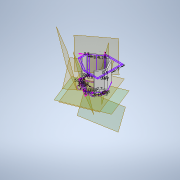
# Autodesk Inventor part: mouse_cam_base_final_withgyro_wall
Saved by Autodesk Inventor 2022 (Build 260153000, 153)
## iProperties
Created: 2022-03-01
Part Number: mouse_cam_base_final_withgyro_wall
Material: Generic
Document SubType Name: Modeling
Designer: Cornell
Density: 1 g/cm^3
Appearance: Default
Author: Cornell
Autodesk Inventor part; units mm, degrees
sketch "Sketch1" plane through (0, 0, 0) normal (0, 1, 0) x (-1, 0, 0)
  line L0 (0, 0) -> (0, 6.2) construction
  line L1 (0, 6.2) -> (10.144349, 0.343157) construction
  line L2 (0, 0) -> (-2.7, 0) construction
  line L3 (-2.7, 0) -> (-2.7, 5.13) construction
  line L4 (-2.7, 5.13) -> (0, 6.2) construction
  line L5 (-2.7, 0) -> (-5.7, 0) construction
  line L6 (-5.7, 0) -> (-2.7, 5.13) construction
  line L7 (-5.7, 0) -> (-6.5, 0)
  line L8 (-6.423049, 0.342344) -> (-3.493848, 5.594239)
  line L9 (0.128209, 7.130954) -> (-3.493848, 5.594239) construction
  line L10 (0.128209, 7.130954) -> (10.551194, 1.035641) construction
  line L11 (10.144349, 0.343157) -> (0, 6.2) construction
  line L12 (-5.7, 0) -> (-2.7, 5.13) construction
  line L13 (0, 6.2) -> (10.144349, 0.343157) construction
  line L14 (10.551194, 1.035641) -> (10.144349, 0.343157) construction
  line L15 (0, 6.2) -> (0.438353, 6.949583)
  line L16 (0.438353, 6.949583) -> (3.02804, 5.435146) construction
  line L17 (3.02804, 5.435146) -> (2.602221, 4.697607) construction
  line L18 (0, 6.2) -> (-0.381289, 6.498511) construction
  line L19 (-0.381289, 6.498511) -> (0.106711, 7.121833) construction
  line L20 (-5.7, 0) -> (-2.7, -5.13) construction
  line L21 (-6.423049, -0.342344) -> (-3.493848, -5.594239)
  line L22 (-6.423049, 0.342344) -> (-6.423049, -0.342344)
  line L23 (-5.559009, 0.241095) -> (-5.559009, -0.241095)
  line L24 (-5.559009, 0) -> (4.440991, 0) construction
  line L25 (-5.559009, 0) -> (5.440991, 0) construction
  line L26 (5.440991, 0) -> (6.440991, 0) construction
  line L27 (5.440991, 0) -> (6.240991, 0)
  line L28 (10.144349, 0.343157) -> (10.144349, -0.005356)
  line L29 (10.144349, -0.005356) -> (10.144349, -0.347701)
  line L30 (10.144349, -0.347701) -> (5.339701, -3.117122) construction
  line L31 (10.551194, 1.035641) -> (10.551194, -1.035641) construction
  line L32 (10.551194, -1.035641) -> (6.240991, -3.556227) construction
  line L33 (5.440991, 0) -> (7.810991, 0) construction
  line L34 (7.810991, 0) -> (7.810991, 1.690322)
  line L35 (7.810991, 0) -> (7.810991, -1.692659)
  line L36 (7.810991, 0) -> (8.610991, 0) construction
  line L37 (8.610991, 0) -> (8.610991, 1.228442)
  line L38 (8.610991, 0) -> (8.610991, -1.231535)
  line L39 (8.610991, -1.231535) -> (8.610991, -2.170262)
  line L40 (7.810991, -1.692659) -> (7.810991, -2.638099)
  line L41 (0, -6.2) -> (0, -4.7)
  line L42 (6.240991, -3.556227) -> (2.598076, -5.686587) construction
  line L43 (-2.951462, -4.7) -> (-5.559009, -0.241095)
  line L44 (-3.493848, -5.594239) -> (-2.951462, -4.7)
  line L45 (-5.559009, 0.241095) -> (-2.951462, 4.7)
  line L46 (10.551194, 1.035641) -> (2.755992, 5.594239) construction
  line L47 (2.602221, 4.697607) -> (10.144349, 0.343157) construction
  line L48 (-5.559009, -0.241095) -> (-5.559009, 0.241095)
  line L49 (-2.951462, 4.7) -> (-3.493848, 5.594239)
  line L50 (-6.423049, -0.342344) -> (-5.559009, -0.241095)
  line L51 (-6.423049, 0.342344) -> (-5.559009, 0.241095)
  line L52 (7.810991, -1.692659) -> (8.610991, -1.231535)
  line L53 (7.810991, 1.690322) -> (8.610991, 1.228442)
  line L54 (8.610991, 1.228442) -> (8.610991, 2.170262)
  line L55 (7.810991, 1.690322) -> (7.810991, 2.638099)
  line L56 (7.810991, 2.638099) -> (8.610991, 2.170262)
  line L57 (2.593853, -4.401195) -> (-2.951462, -4.7)
  line L58 (-3.493848, -5.594239) -> (2.69542, -5.260734)
  line L59 (2.593853, -4.401195) -> (8.610991, -1.231535)
  line L60 (2.69542, -5.260734) -> (8.610991, -2.170262)
  line L61 (2.593853, -4.401195) -> (2.69542, -5.260734)
  line L62 (2.593853, 4.401195) -> (-2.951462, 4.7)
  line L63 (-3.493848, 5.594239) -> (2.69542, 5.260734)
  line L64 (2.593853, 4.401195) -> (2.69542, 5.260734)
  line L65 (-2.951462, 4.7) -> (2.593853, 4.401195)
  line L66 (2.644637, 4.830965) -> (2.69542, 5.260734)
  line L67 (-3.493848, 5.594239) -> (-2.951462, 4.7)
  point P0 (2.602221, 4.697607)
  point P1 (-5.29708, 0.688993)
  dimension "d0" = 6.2
  dimension "d1" = 60
  dimension "d2" = 2.7
  dimension "d3" = 5.13
  dimension "d4" = 3
  dimension "d7" = 0.8
  dimension "d8" = 0.8
  dimension "d20" = 3
  dimension "d33" = 10
  dimension "d36" = 0.8
  dimension "d73" = 2.37
  dimension "d74" = 0.8
  constraints: 136 end point, 28 point on line, 14 collinear, 7 perpendicular, 7 symmetric about line, 4 parallel, 4 vertical, 3 horizontal, 2 midpoint
  measures "d0" distance of L0.start L0.end
  measures "d1" angle of L0 L1
  measures "d2" distance of L0.start L2.end
  measures "d3" distance of L2.end L3.end
  measures "d4" distance of L2.end L5.end
  measures "d7" distance of L5.end L7.end
  measures "d8" distance of L5.end L8.start
  measures "d20" distance of L15.end L16.end
  measures "d33" distance of L24.start L24.end
  measures "d36" distance of L25.end L27.end
  measures "d73" distance of L25.end L33.end
  measures "d74" distance of L33.end L36.end
ref_plane "Work Plane1" through (2.7, 0, 5.13) normal (0, 1, 0) x (-0.9296593, 0, 0.3684205)
ref_plane "Work Plane2" through (2.7, 3, 5.13) normal (0, 1, 0) x (-0.9296593, 0, 0.3684205)
sketch "Sketch2" plane through (2.7, 3, 5.13) normal (0, 1, 0) x (-0.9296593, 0, 0.3684205)
  line L0 (-5.025918, -0.734007) -> (-6.376038, -1.814103)
  line L1 (-5.876282, -2.438798) -> (-1.068891, 1.407115)
  line L2 (3.395875, 2.207115) -> (-1.349515, 2.207115)
  line L3 (-1.349515, 2.207115) -> (-5.025918, -0.734007)
  line L4 (0.620083, -5.763887) -> (-1.890319, -4.77089) construction
  line L5 (-6.938992, -5.570456) -> (-7.184919, -3.859038)
  line L6 (-6.393053, -3.745249) -> (-5.517376, -9.839118)
  line L7 (-5.517376, -9.839118) -> (-2.260723, -12.893351)
  line L8 (-2.260723, -12.893351) -> (-2.807982, -13.476881)
  line L9 (-2.807982, -13.476881) -> (-6.269327, -10.230679)
  line L10 (-6.269327, -10.230679) -> (-6.938992, -5.570456)
  line L11 (-5.876282, -2.438798) -> (-6.393053, -3.745249)
  line L12 (-7.184919, -3.859038) -> (-6.376038, -1.814103)
  line L13 (-2.260723, -12.893351) -> (-1.956037, -13.211044)
  line L14 (-2.807982, -13.476881) -> (-2.146425, -14.097318)
  line L15 (6.305657, -10.853277) -> (-1.956037, -13.211044)
  line L16 (6.901194, -11.51526) -> (-2.146425, -14.097318)
  line L17 (-1.349515, 2.207115) -> (-2.349515, 1.407115)
  line L18 (-5.646461, -8.940808) -> (-6.438327, -9.054598)
  line L19 (6.901194, -11.51526) -> (7.800754, -11.250894)
  line L20 (6.667165, -11.582048) -> (8.800527, -6.188688)
  line L21 (7.800754, -11.250894) -> (9.479308, -7.007336)
  line L22 (6.305657, -10.853277) -> (8.171706, -10.31309)
  line L23 (9.451627, -6.973952) -> (9.479308, -7.007336)
  line L24 (9.479308, -7.007336) -> (9.191715, -7.734401)
  line L25 (9.191715, -7.734401) -> (9.479308, -7.007336)
  line L26 (9.479308, -7.007336) -> (8.800527, -6.188688)
  line L27 (-1.068891, 1.407115) -> (-1.349515, 2.207115)
  line L28 (4.0365, -0.443004) -> (3.982037, -0.377319)
  line L29 (-5.876282, -2.438798) -> (-1.068891, 1.407115)
  line L30 (-1.068891, 1.407115) -> (3.395875, 1.407115)
  line L31 (3.395875, 1.407115) -> (3.395875, 2.207115)
  line L32 (3.395875, 2.207115) -> (-1.349515, 2.207115)
  line L33 (-1.349515, 2.207115) -> (-5.025918, -0.734007)
  line L34 (8.171706, -10.31309) -> (7.238681, -10.137195)
  line L35 (6.667165, -11.582048) -> (6.444559, -10.813068)
  line L36 (-1.956037, -13.211044) -> (-1.475233, -13.073829)
  line L37 (-1.475233, -13.073829) -> (-1.25569, -13.843115)
  point P0 (10.376244, -11.325229)
  point P1 (8.145173, -8.377747)
  point P2 (-1.849759, 0.78242)
  point P3 (8.512934, -6.915753)
  dimension "d14" = 0.8
  dimension "d191" = 0.5
  constraints: 76 end point, 16 point on line, 7 symmetric about line, 4 perpendicular, 3 parallel, 2 collinear
  measures "d14" distance of L0.end L1.start
  measures "d191" distance of L13.end L36.end
sketch "Sketch3" plane through (2.7, 3, 5.13) normal (0, 1, 0) x (-0.9296593, 0, 0.3684205)
  line L0 (2.486687, 1.818535) -> (1.814017, 1.280761)
  line L1 (2.486687, 1.818535) -> (8.984898, -6.309695)
  line L2 (8.984898, -6.309695) -> (9.36787, -6.788734)
  line L3 (8.466395, -7.040307) -> (8.167217, -7.782259)
  line L4 (8.167217, -7.782259) -> (9.054862, -8.087151)
  line L5 (9.054862, -8.087151) -> (9.495491, -6.948366)
  line L6 (2.486687, 1.818535) -> (9.495491, -6.948366)
  line L7 (8.466395, -7.040307) -> (1.814017, 1.280761)
  point P0 (0.620083, -5.763887)
  point P1 (9.36787, -6.788734)
  point P2 (8.984898, -6.309695)
  dimension "d166" = 0.8
  constraints: 16 end point, 1 collinear
  measures "d166" distance of L3.start L3.end
ref_plane "Work Plane5" through (2.7, 0, 5.13) normal (-0.3335527, 0.4246479, -0.841675) x (-0.8367361, 0.2779443, 0.4718259)
sketch "Sketch4" plane through (2.7, 0, 5.13) normal (-0.3335527, 0.4246479, -0.841675) x (-0.8367361, 0.2779443, 0.4718259)
  line L0 (1.996279, 2.105742) -> (1.587489, 0.879372)
  line L1 (1.587489, 0.879372) -> (0.871772, 1.117944)
  line L2 (0.871772, 1.117944) -> (1.294635, 2.386534)
  line L3 (1.294635, 2.386534) -> (2.176917, 2.09244)
  point P0 (-0.161279, -2.519791)
  constraints: 8 end point, 3 perpendicular
ref_plane "Work Plane3" through (2.933487, -0.297253, 5.719172) normal (-0.3335527, 0.4246479, -0.841675) x (-0.8367361, 0.2779443, 0.4718259)
sketch "Sketch5" plane through (2.7, 3, 5.13) normal (0, 1, 0) x (-0.9296593, 0, 0.3684205)
  line L0 (-5.876282, -2.438798) -> (-1.068891, 1.407115)
  line L1 (-1.820829, 0.805564) -> (-2.307957, 1.414474)
  line L2 (-7.184919, -3.859038) -> (-6.269327, -10.230679)
  line L3 (-2.307957, 1.414474) -> (-1.350688, 2.180289)
  line L4 (-1.383047, 2.180289) -> (-6.376038, -1.814103)
  line L5 (3.395875, 1.710746) -> (3.395875, 2.180289)
  line L6 (-1.350688, 2.180289) -> (3.395875, 2.180289)
  line L7 (3.395875, 2.180289) -> (3.395875, 1.407115)
  line L8 (3.395875, 1.407115) -> (-1.068891, 1.407115)
  line L9 (-3.779995, -9.538304) -> (-5.517376, -9.839118)
  line L10 (-2.249693, -12.903695) -> (-5.517376, -9.839118)
  line L11 (-5.517376, -9.839118) -> (-5.741278, -8.280977)
  line L12 (-5.741278, -8.280977) -> (-5.517376, -9.839118)
  line L13 (-1.854009, -11.349234) -> (-2.260723, -12.893351)
  line L14 (6.901194, -11.51526) -> (8.942661, -6.366356)
  line L15 (3.322414, 0.773174) -> (9.366764, -6.78735)
  line L16 (2.815603, 1.407115) -> (2.815603, 1.407115)
  line L17 (2.815603, 1.407115) -> (2.815603, 1.407115)
  line L18 (2.486687, 1.818535) -> (9.366764, -6.78735)
  line L19 (2.815603, 1.407115) -> (3.395875, 2.180289)
  line L20 (2.815603, 1.407115) -> (2.815603, 1.407115)
  line L21 (8.693313, -7.325747) -> (1.813236, 1.280137)
  point P0 (0.620083, -5.763887)
  point P1 (8.984899, -6.309695)
  point P2 (1.814017, 1.280761)
  point P3 (8.311447, -6.848094)
  constraints: 26 end point, 4 perpendicular, 4 point on line, 2 collinear, 1 parallel, 2 other
ref_plane "Work Plane4" through (2.7, 16, 5.13) normal (0, 1, 0) x (-0.9296593, 0, 0.3684205)
sketch "Sketch6" plane through (2.7, 16, 5.13) normal (0, 1, 0) x (-0.9296593, 0, 0.3684205)
  line L0 (-9.395095, -1.714761) -> (-12.713432, -10.080683)
  line L1 (-6.065575, 6.679353) -> (-9.395095, -1.714761)
  line L2 (1.902995, -15.875887) -> (2.197853, -15.132208) construction
  line L3 (-11.651687, -9.573329) -> (-5.617763, 5.645188)
  line L4 (-5.617763, 5.645188) -> (2.374332, 2.396864)
  line L5 (-6.065575, 6.679353) -> (2.726743, 3.105785)
  line L6 (-5.617763, 5.645188) -> (-6.065575, 6.679353)
  line L7 (-12.713432, -10.080683) -> (-11.651687, -9.573329)
  line L8 (-1.057302, -14.702172) -> (-12.713432, -10.080683)
  line L9 (-0.827268, -13.865057) -> (-11.651687, -9.573329)
  line L10 (2.374332, 2.396864) -> (3.085093, 2.927646)
  line L11 (2.726743, 3.105785) -> (3.085093, 2.927646)
  line L12 (8.370103, -7.808325) -> (9.110242, -8.111959)
  line L13 (9.110242, -8.111959) -> (9.948329, -6.111694)
  line L14 (9.110242, -8.111959) -> (7.808238, -11.245281)
  line L15 (8.370103, -7.808325) -> (7.167218, -10.740485)
  line L16 (7.808238, -11.245281) -> (8.0001, -10.783557)
  line L17 (8.0001, -10.783557) -> (7.310858, -10.390347)
  line L18 (7.167218, -10.740485) -> (6.492259, -10.988462)
  line L19 (6.665132, -11.579582) -> (6.492259, -10.988462)
  line L20 (7.808238, -11.245281) -> (6.688123, -11.658198)
  line L21 (6.688123, -11.658198) -> (6.492259, -10.988462)
  line L22 (-1.145334, -14.667268) -> (-0.827268, -13.865057)
  line L23 (8.984899, -6.309695) -> (8.370103, -7.808325)
  line L24 (8.984899, -6.309695) -> (2.374332, 2.396864)
  line L25 (9.948329, -6.111694) -> (3.085093, 2.927646)
  line L26 (8.984899, -6.309695) -> (9.691387, -5.773285)
  line L27 (6.829738, -10.864473) -> (7.070388, -11.517281)
  point P0 (9.042998, -8.114904)
  point P1 (9.054862, -8.087151)
  point P2 (6.665132, -11.579582)
  dimension "d44" = 9
  dimension "d182" = 0.5
  constraints: 56 end point, 6 point on line, 4 perpendicular, 3 parallel, 2 collinear, 1 midpoint
  measures "d44" distance of L0.start L0.end
  measures "d182" distance of L14.end L16.end
ref_plane "Work Plane10" through (2.7, 0, 5.13) normal (0, -1, 0) x (0.9296593, 0, -0.3684205)
sketch "Sketch12" plane through (2.7, 0, 5.13) normal (0, -1, 0) x (0.9296593, 0, -0.3684205)
  line L0 (4.636726, -3.939971) -> (4.459077, -3.491698)
  line L1 (4.547901, -3.715834) -> (-6.244742, -7.994963)
  line L2 (-11.636416, -10.132685) -> (-11.330506, -10.904239)
  line L3 (-6.244742, -7.994963) -> (-11.636416, -10.132685)
  line L4 (-11.636416, -10.132685) -> (-9.265961, -7.13977)
  line L5 (-11.636416, -10.132685) -> (-7.818485, -10.132685) construction
  line L6 (-9.265961, -7.13977) -> (-5.70436, -2.206262)
  line L7 (-9.366764, -6.78735) -> (-2.815603, 1.407115)
  line L8 (-6.244742, -7.994963) -> (-7.48516, -4.673016)
  circle A0 centre (-7.48516, -4.673016) radius 2.31
  line L9 (-8.499293, -7.08306) -> (-2.218533, 0.773174)
  line L10 (-1.303832, -11.09047) -> (-0.840832, -10.906985)
  point P0 (-0.620083, -5.763887)
  point P1 (-4.119299, -0.223603)
  point P2 (-4.696345, -2.326175)
  point P3 (-8.693313, -7.325747)
  point P4 (-2.486687, 1.818536)
  dimension "d158" = 11.61
  dimension "d159" = 5.8
  dimension "d161" = 51.62
  dimension "d162" = 4.62
  constraints: 14 end point, 2 midpoint, 1 centre point, 1 coincident, 1 equal length, 1 horizontal, 1 perpendicular, 1 point on line
  measures "d158" distance of L1.start L1.end
  measures "d159" distance of L1.end L2.start
  measures "d161" angle of L5 L4
  measures "d162" diameter of A0
ref_plane "Work Plane9" through (-7.958217, 3, -3.032726) normal (0, 1, 0) x (0.7928621, 0, -0.6094011)
sketch "Sketch13" plane through (-7.958217, 3, -3.032726) normal (0, 1, 0) x (0.7928621, 0, -0.6094011)
  line L0 (-0.937573, -0.007351) -> (-3.009709, -2.706893)
  line L1 (-0.937573, -0.007351) -> (-1.242019, -0.403978)
  line L2 (-1.242019, -0.403978) -> (-0.502458, -0.971656)
  line L3 (-2.244126, -3.240669) -> (-0.372916, -0.802891)
  line L4 (-0.372916, -0.802891) -> (0.391006, -0.8)
  line L5 (-0.502458, -0.971656) -> (-0.372916, -0.802891)
  line L6 (-0.372916, -0.802891) -> (0.12708, -0.800999)
  line L7 (0.12708, -0.800999) -> (0.124046, 0.000973)
  line L8 (0, 0) -> (-0.937573, -0.007351)
  line L9 (0.124046, 0.000973) -> (-0.937573, -0.007351)
  point P0 (4.461622, -7.25428)
  dimension "d183" = 0.5
  dimension "d184" = 0.5
  constraints: 12 end point, 3 point on line, 2 perpendicular, 1 collinear
  measures "d183" distance of L0.start L1.end
  measures "d184" distance of L3.end L6.end
sketch "Sketch6 outline for Extrusion4" plane through (2.7, 16, 5.13) normal (0, 1, 0) x (-0.9296593, 0, 0.3684205)
  line L0 (9.110242, -8.111959) -> (8.370103, -7.808325)
  line L1 (8.0001, -10.783557) -> (9.110242, -8.111959)
  line L2 (7.310858, -10.390347) -> (8.0001, -10.783557)
  line L3 (8.370103, -7.808325) -> (7.310858, -10.390347)
extrude "Extrusion4" add sketch "Sketch6 outline for Extrusion4" against normal blind 13
ref_plane "Work Plane8" through (2.7, 3, 5.13) normal (0, 1, 0) x (0.9296593, 0, -0.3684205)
sketch "Sketch15" plane through (2.7, 3, 5.13) normal (0, 1, 0) x (0.9296593, 0, -0.3684205)
  line L0 (1.956037, 13.211044) -> (2.260723, 12.893351)
  line L1 (2.2586, 12.895565) -> (1.956037, 13.211044)
  line L2 (1.956037, 13.211044) -> (1.469205, 13.072109)
  line L3 (1.249662, 13.841395) -> (1.469205, 13.072109)
  line L4 (1.249662, 13.841395) -> (2.146425, 14.097318)
  line L5 (2.805748, 13.478976) -> (2.146425, 14.097318)
  line L6 (6.269327, 10.230679) -> (6.360384, 9.597006)
  line L7 (5.517376, 9.839118) -> (5.014673, 10.310575)
  line L8 (2.260723, 12.893351) -> (5.517376, 9.839118)
  line L9 (5.561933, 10.894104) -> (6.269327, 10.230679)
  line L10 (6.360384, 9.597006) -> (6.269327, 10.230679)
  line L11 (5.517376, 9.839118) -> (6.393053, 3.745249)
  line L12 (5.609766, 9.196174) -> (5.517376, 9.839118)
  line L13 (5.517376, 9.839118) -> (5.014673, 10.310575)
  line L14 (5.561933, 10.894104) -> (2.805748, 13.478976)
  line L15 (-0.937465, 10.652712) -> (2.260723, 12.893351)
  line L16 (2.260723, 12.893351) -> (5.014673, 10.310575)
  line L17 (7.184919, 3.859038) -> (6.269327, 10.230679)
  line L18 (6.360384, 9.597006) -> (7.184919, 3.859038)
  line L19 (5.225038, 3.079241) -> (6.376038, 1.814103)
  line L20 (7.184919, 3.859038) -> (6.376038, 1.814103)
  line L21 (6.376038, 1.814103) -> (1.373089, -2.224092)
  line L22 (1.373089, -2.224092) -> (-2.323998, -2.207115)
  line L23 (-3.395875, -2.207115) -> (1.349515, -2.207115)
  line L24 (-2.374332, -2.396864) -> (-1.814017, -1.280761)
  line L25 (0.392195, 0.30711) -> (1.068891, -1.407115)
  line L26 (-1.87745, -1.407115) -> (1.068891, -1.407115)
  line L27 (1.068891, -1.407115) -> (5.896292, 2.489385)
  line L28 (5.896292, 2.489385) -> (6.393053, 3.745249)
  line L29 (-1.972065, -1.407115) -> (-1.814017, -1.280761)
  line L30 (-3.395875, -2.207115) -> (-1.972065, -1.407115)
  line L31 (1.349515, -2.207115) -> (6.376038, 1.814103)
  line L32 (2.260723, -1.478149) -> (1.698044, -0.903792)
  line L33 (5.876282, 2.438798) -> (1.068891, -1.407115)
  point P0 (-0.620083, 5.763887)
  point P1 (5.83659, 2.407044)
  point P2 (5.561933, 10.894104)
  point P3 (5.818675, 2.426736)
  constraints: 44 end point, 6 collinear, 5 point on line, 2 parallel, 1 horizontal, 1 perpendicular
ref_plane "Work Plane11" through (-2.344891, 5.121654, 5.755597) normal (0.4993148, 0.2017185, -0.8426117) x (-0.8599057, -0.0036627, -0.5104397)
ref_plane "Work Plane12" through (-14.166609, 14.001501, 5.586149) normal (-0.4993148, -0.2017185, 0.8426117) x (0.8599057, 0.0036627, 0.5104397)
sketch "Sketch18" plane through (-14.166609, 14.001501, 5.586149) normal (-0.4993148, -0.2017185, 0.8426117) x (0.8599057, 0.0036627, 0.5104397)
  line L0 (-2.976562, 0.79375) -> (-2.976562, 2.182813)
  line L1 (-2.976562, 1.488281) -> (0, 1.488281)
  line L2 (0, 0) -> (0, 2.182813)
  line L3 (-2.182812, 2.976563) -> (-0.79375, 2.976563)
  line L4 (-1.488281, 2.976563) -> (-1.488281, 0)
  line L5 (-2.182812, 0) -> (0, 0)
  point P0 (9.279272, -16.174723)
  point P1 (-1.488281, 1.488281)
  constraints: 4 end point, 3 midpoint, 2 point on line, 1 horizontal, 1 perpendicular
hole "Hole3" [suppressed]
ref_plane "Work Plane6" through (-4.067068, 16, -5.128768) normal (0.5917808, 0.0071089, 0.8060676) x (-0.0120118, 0.9999279, 0)
sketch "Sketch19" plane through (-4.067068, 16, -5.128768) normal (0.5917808, 0.0071089, 0.8060676) x (-0.0120118, 0.9999279, 0)
  line L0 (0.000015, -0.00049) -> (0.045215, -4.200247)
  line L1 (0.045215, -4.200247) -> (0.040608, 4.199752)
  line L2 (0.046282, 4.830336) -> (0.039842, 4.114612)
  line L3 (0.040608, 4.199752) -> (0.040608, 4.199752)
  line L4 (-0.042867, -5.029352) -> (-0.033986, -4.097053)
  line L5 (-13.04043, -4.746024) -> (-13.030903, -3.746069)
  line L6 (0.000015, -0.00049) -> (-12.995218, -0.00049)
  line L7 (-13.04043, 4.745044) -> (-13.030903, 3.745089)
  line L8 (-13.04043, 4.745044) -> (-13.030903, 3.745089)
  line L9 (0.056854, 8.692866) -> (-0.049679, 4.719917)
  line L10 (-0.040168, -4.746138) -> (0.045514, -4.746091)
  line L11 (-0.040168, -4.746024) -> (-0.040168, -4.246024)
  line L12 (-0.040168, -4.746024) -> (0.044968, -3.749655)
  line L13 (0.044968, -3.749655) -> (-13.030903, -3.746069)
  line L14 (-13.04043, -4.746024) -> (-13.030903, -3.746069)
  line L15 (-13.04043, 4.745044) -> (-13.04043, -4.746091)
  line L16 (0.045514, -4.746091) -> (0.045514, 4.745044)
  line L17 (0.045514, 4.745044) -> (0.045514, 3.745044)
  line L18 (0.045514, 3.745044) -> (-13.030903, 3.745089)
  line L19 (-13.030903, 3.745089) -> (-13.008011, 4.746098)
  line L20 (-13.030903, -3.746069) -> (-13.044212, -4.545959)
  line L21 (-13.044212, -4.545959) -> (0.045514, -4.5465)
  line L22 (-12.959539, 3.745089) -> (-13.012648, 4.543324)
  line L23 (-13.012648, 4.543324) -> (-0.037961, 4.543324)
  line L24 (-0.052606, 3.997168) -> (0.046972, 7.710746)
  line L25 (0.045514, 4.543324) -> (-0.037961, 4.543324)
  line L26 (-3.974868, -4.546334) -> (-3.97465, -3.748552)
  line L27 (-9.023068, -3.747168) -> (-9.023101, -4.546125)
  line L28 (-3.972595, 3.745058) -> (-3.972376, 4.543324)
  line L29 (-9.022758, 3.745075) -> (-9.022725, 4.543324)
  line L30 (-13.030903, -3.746069) -> (-12.959539, 3.745089)
  line L31 (-12.961902, 4.094208) -> (-13.043726, -4.494865)
  line L32 (-12.995218, -0.00049) -> (-12.981812, 1.407042)
  line L33 (-12.981812, 1.407042) -> (-13.008941, -1.440706)
  line L34 (-13.008941, -1.440706) -> (-12.47059, -1.440706)
  line L35 (-12.47059, -1.440706) -> (-12.44351, 1.401914)
  line L36 (-12.44351, 1.401914) -> (-12.981812, 1.407042)
  point P0 (-16.047699, -0.087853)
  point P1 (-13.038524, -4.545959)
  point P2 (-0.023119, -4.546497)
  point P3 (-13.038524, -4.545959)
  point P4 (-0.040168, -4.546497)
  point P5 (0.043699, 4.543324)
  point P6 (0.040857, 3.745044)
  point P7 (-13.04043, -4.318645)
  point P8 (0.04088, -3.797492)
  point P9 (0.040365, -3.749653)
  dimension "d221" = 4.2
  dimension "d222" = 8.4
  dimension "d223" = 1
  dimension "d231" = 0.5
  dimension "d232" = 1
  dimension "d233" = 1
  dimension "d236" = 0.8
  dimension "d237" = 0.8
  constraints: 64 end point, 24 point on line, 4 perpendicular, 2 horizontal, 2 parallel, 2 symmetric about line, 2 vertical, 1 collinear
  measures "d221" distance of L0.start L0.end
  measures "d222" distance of L0.end L1.end
  measures "d223" distance of L5.start L5.end
  measures "d231" distance of L11.start L11.end
  measures "d232" distance of L11.start L12.end
  measures "d233" distance of L16.end L17.end
  measures "d236" distance of L5.end L20.end
  measures "d237" distance of L22.start L22.end
ref_plane "Work Plane7" through (-2.666496, 2.984981, -9.763999) normal (-0.806088, 0, 0.5917957) x (0.5917808, 0.0071089, 0.8060676)
sketch "Sketch21" plane through (-2.666496, 2.984981, -9.763999) normal (-0.806088, 0, 0.5917957) x (0.5917808, 0.0071089, 0.8060676)
  line L0 (2.11273, 0) -> (0, 0)
  line L1 (0, 0) -> (0.5, 0)
  line L2 (0.5, 0) -> (0.5, 12.991344)
  line L3 (2.202954, 12.991344) -> (0, 12.991344)
  line L4 (0.5, 12.991344) -> (0, 12.991344)
  line L5 (0, 12.999808) -> (0, 0.021767)
  line L6 (2.090892, 0.021767) -> (0, 0.021767)
  line L7 (0, 0.021767) -> (0, 0)
  line L8 (0, 0) -> (0, 0.021767)
  point P0 (9.427205, -3.052075)
  point P1 (0.5, 0.021767)
  point P2 (0, 12.991344)
  dimension "d226" = 0.5
  constraints: 10 end point, 2 point on line, 1 collinear, 1 horizontal, 1 perpendicular, 1 vertical
  measures "d226" distance of L0.end L1.end
sketch "Sketch19 outline for Extrusion9" plane through (-4.067068, 16, -5.128768) normal (0.5917808, 0.0071089, 0.8060676) x (-0.0120118, 0.9999279, 0)
  line L0 (-9.023068, -3.747168) -> (-9.023101, -4.546125)
  line L1 (-3.97465, -3.748552) -> (-9.023068, -3.747168)
  line L2 (-3.974868, -4.546334) -> (-3.97465, -3.748552)
  line L3 (-9.023101, -4.546125) -> (-3.974868, -4.546334)
extrude "Extrusion9" add sketch "Sketch19 outline for Extrusion9" against normal blind 3.5
sketch "Sketch19 outline for Extrusion11" plane through (-4.067068, 16, -5.128768) normal (0.5917808, 0.0071089, 0.8060676) x (-0.0120118, 0.9999279, 0)
  line L0 (-9.022725, 4.543324) -> (-9.022758, 3.745075)
  line L1 (-3.972376, 4.543324) -> (-9.022725, 4.543324)
  line L2 (-3.972595, 3.745058) -> (-3.972376, 4.543324)
  line L3 (-9.022758, 3.745075) -> (-3.972595, 3.745058)
extrude "Extrusion11" add sketch "Sketch19 outline for Extrusion11" against normal blind 3.5
sketch "Sketch22" plane through (-0.891176, 3.006307, -7.34578) normal (-0.8060127, -0.0094082, 0.5918234) x (0.5917808, 0.0071089, 0.8060676)
  line L0 (-3.5, 0) -> (-3, 0)
  line L1 (-3.5, 4.007835) -> (-3.5, 9.056254)
  line L2 (-3.5, 13.075872) -> (-3, 13.075872)
  line L3 (-3, 13.075872) -> (-3, 0)
  line L4 (-3.5, 0) -> (-3.5, 13.075872)
  line L5 (-3.5, 13.075872) -> (-3.5, 0)
  line L6 (-3, 0) -> (-3.5, 0)
  line L7 (0, 9.056254) -> (-3.5, 9.056254)
  line L8 (-3.5, 9.056254) -> (-3, 9.056254)
  line L9 (0, 4.008021) -> (-3.5, 4.008021)
  line L10 (-3.5, 4.008021) -> (-3, 4.008021)
  point P0 (6.427205, -3.017798)
  point P1 (-3.5, 4.007835)
  dimension "d240" = 0.5
  dimension "d241" = 0.5
  constraints: 16 end point, 4 point on line, 1 collinear, 1 perpendicular
  measures "d240" distance of L0.start L0.end
  measures "d241" distance of L2.start L2.end
sketch "Sketch23" plane through (-6.93042, 3.041956, -2.912337) normal (0.8060095, 0.0096789, -0.5918235) x (-0.5917808, -0.0071089, -0.8060676)
  line L0 (3.5, 8.95012) -> (3.5, 3.899957)
  line L1 (3.5, 12.963572) -> (3, 12.963572)
  line L2 (3, 12.963572) -> (3, 0)
  line L3 (3, 0) -> (3.5, 0)
  line L4 (3.5, 0) -> (3.5, 12.963572)
  line L5 (0, 8.95012) -> (3.5, 8.95012)
  line L6 (3, 8.95012) -> (3.5, 8.95012)
  line L7 (0, 3.899987) -> (3.5, 3.899987)
  line L8 (3, 3.899987) -> (3.5, 3.899987)
  point P0 (-6.427205, -3.124971)
  point P1 (3.5, 0)
  point P2 (3.5, 0)
  point P3 (3.5, 3.899957)
  dimension "d244" = 0.5
  constraints: 12 end point, 4 point on line, 3 perpendicular, 2 collinear, 1 horizontal
  measures "d244" distance of L1.start L1.end
sketch "Sketch19 outline for Extrusion14" plane through (-4.067068, 16, -5.128768) normal (0.5917808, 0.0071089, 0.8060676) x (-0.0120118, 0.9999279, 0)
  line L0 (-13.030903, -3.746069) -> (0.044968, -3.749655)
  line L1 (-13.04043, -4.318645) -> (-13.030903, -3.746069)
  line L2 (-13.04043, 4.745044) -> (-13.04043, -4.318645)
  line L3 (-13.030903, 3.745089) -> (-13.04043, 4.745044)
  line L4 (0.040857, 3.745044) -> (-13.030903, 3.745089)
  line L5 (0.044968, -3.749655) -> (0.040857, 3.745044)
extrude "Extrusion14" add sketch "Sketch19 outline for Extrusion14" against normal blind 0.8
sketch "Sketch19 outline for Extrusion15" plane through (-4.067068, 16, -5.128768) normal (0.5917808, 0.0071089, 0.8060676) x (-0.0120118, 0.9999279, 0)
  line L0 (-12.44351, 1.401914) -> (-12.981812, 1.407042)
  line L1 (-12.47059, -1.440706) -> (-12.44351, 1.401914)
  line L2 (-13.008941, -1.440706) -> (-12.47059, -1.440706)
  line L3 (-12.981812, 1.407042) -> (-13.008941, -1.440706)
extrude "Extrusion15" add sketch "Sketch19 outline for Extrusion15" against normal blind 3.5
sketch "Sketch22 outline for Extrusion16" plane through (-0.891176, 3.006307, -7.34578) normal (-0.8060127, -0.0094082, 0.5918234) x (0.5917808, 0.0071089, 0.8060676)
  line L0 (-3.5, 4.008021) -> (-3, 4.008021)
  line L1 (-3.5, 9.056254) -> (-3.5, 4.008021)
  line L2 (-3, 9.056254) -> (-3.5, 9.056254)
  line L3 (-3, 4.008021) -> (-3, 9.056254)
extrude "Extrusion16" add sketch "Sketch22 outline for Extrusion16" along normal blind 0.5
sketch "Sketch23 outline for Extrusion17" plane through (-6.93042, 3.041956, -2.912337) normal (0.8060095, 0.0096789, -0.5918235) x (-0.5917808, -0.0071089, -0.8060676)
  line L0 (3, 3.899987) -> (3.5, 3.899987)
  line L1 (3, 8.95012) -> (3, 3.899987)
  line L2 (3.5, 8.95012) -> (3, 8.95012)
  line L3 (3.5, 3.899987) -> (3.5, 8.95012)
extrude "Extrusion17" add sketch "Sketch23 outline for Extrusion17" along normal blind 0.5
sketch "Sketch19 outline for Extrusion18" plane through (-4.067068, 16, -5.128768) normal (0.5917808, 0.0071089, 0.8060676) x (-0.0120118, 0.9999279, 0)
  line L0 (-9.022758, 3.745075) -> (-9.022725, 4.543324)
  line L1 (-12.959539, 3.745089) -> (-9.022758, 3.745075)
  line L2 (-13.012648, 4.543324) -> (-12.959539, 3.745089)
  line L3 (-9.022725, 4.543324) -> (-13.012648, 4.543324)
  line L4 (-3.972376, 4.543324) -> (-3.972595, 3.745058)
  line L5 (-3.972595, 3.745058) -> (0.040857, 3.745044)
  line L6 (0.040857, 3.745044) -> (0.040608, 4.199752)
  line L7 (0.040608, 4.199752) -> (0.043699, 4.543324)
  line L8 (0.043699, 4.543324) -> (-3.972376, 4.543324)
  line L9 (-9.023101, -4.546125) -> (-9.023068, -3.747168)
  line L10 (-13.038524, -4.545959) -> (-9.023101, -4.546125)
  line L11 (-13.030903, -3.746069) -> (-13.038524, -4.545959)
  line L12 (-9.023068, -3.747168) -> (-13.030903, -3.746069)
  line L13 (-3.97465, -3.748552) -> (-3.974868, -4.546334)
  line L14 (0.040365, -3.749653) -> (-3.97465, -3.748552)
  line L15 (0.04088, -3.797492) -> (0.040365, -3.749653)
  line L16 (-0.023119, -4.546497) -> (0.04088, -3.797492)
  line L17 (-3.974868, -4.546334) -> (-0.023119, -4.546497)
extrude "Extrusion18" add sketch "Sketch19 outline for Extrusion18" against normal blind 0.8
sketch "Sketch6 outline for Extrusion19" plane through (2.7, 16, 5.13) normal (0, 1, 0) x (-0.9296593, 0, 0.3684205)
  line L0 (7.167218, -10.740485) -> (6.492259, -10.988462)
  line L1 (6.492259, -10.988462) -> (6.688123, -11.658198)
  line L2 (6.688123, -11.658198) -> (7.808238, -11.245281)
  line L3 (7.808238, -11.245281) -> (8.0001, -10.783557)
  line L4 (8.0001, -10.783557) -> (7.310858, -10.390347)
  line L5 (7.310858, -10.390347) -> (7.167218, -10.740485)
extrude "Extrusion19" add sketch "Sketch6 outline for Extrusion19" against normal blind 13
sketch "Sketch15 outline for Extrusion20" plane through (2.7, 3, 5.13) normal (0, 1, 0) x (0.9296593, 0, -0.3684205)
  line L0 (5.83659, 2.407044) -> (1.698044, -0.903792)
  line L1 (5.818675, 2.426736) -> (5.83659, 2.407044)
  line L2 (5.896292, 2.489385) -> (5.818675, 2.426736)
  line L3 (6.393053, 3.745249) -> (5.896292, 2.489385)
  line L4 (5.517376, 9.839118) -> (6.393053, 3.745249)
  line L5 (5.014673, 10.310575) -> (5.517376, 9.839118)
  line L6 (2.260723, 12.893351) -> (5.014673, 10.310575)
  line L7 (1.956037, 13.211044) -> (2.260723, 12.893351)
  line L8 (1.469205, 13.072109) -> (1.956037, 13.211044)
  line L9 (1.249662, 13.841395) -> (1.469205, 13.072109)
  line L10 (2.146425, 14.097318) -> (1.249662, 13.841395)
  line L11 (2.805748, 13.478976) -> (2.146425, 14.097318)
  line L12 (5.561933, 10.894104) -> (2.805748, 13.478976)
  line L13 (6.269327, 10.230679) -> (5.561933, 10.894104)
  line L14 (6.360384, 9.597006) -> (6.269327, 10.230679)
  line L15 (7.184919, 3.859038) -> (6.360384, 9.597006)
  line L16 (6.376038, 1.814103) -> (7.184919, 3.859038)
  line L17 (2.260723, -1.478149) -> (6.376038, 1.814103)
  line L18 (1.698044, -0.903792) -> (2.260723, -1.478149)
extrude "Extrusion20" add sketch "Sketch15 outline for Extrusion20" along normal blind 13
body "Solid1"
body "Solid2"
